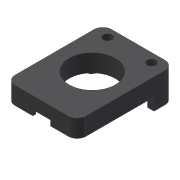
# Autodesk Inventor part: linact_palm_front
Saved by Autodesk Inventor 2014 (Build 180170000, 170)
## iProperties
Created: 2015-05-24
Part Number: linact_palm_front
Material: Generic
Document SubType Name: Modeling
Designer: Martin
Density: 1 g/cm^3
Appearance: Default
Author: Martin
Autodesk Inventor part; units mm, degrees
ref_plane "YZ Plane" through (0, 0, 0) normal (1, 0, 0) x (0, 1, 0)
ref_plane "XZ Plane" through (0, 0, 0) normal (0, 1, 0) x (-1, 0, 0)
sketch "sk_main" plane through (0, 0, 0) normal (0, 0, 1) x (1, 0, 0)
  arc A0 (-6.075, -0.5) -> (-8.075, -2.5) centre (-6.075, -2.5) ccw projected
  line L0 (-8.075, -20.5) -> (-8.075, -2.5) projected
  arc A1 (-8.075, -20.5) -> (-6.075, -22.5) centre (-6.075, -20.5) ccw projected
  line L1 (-6.075, -22.5) -> (6.075, -22.5) projected
  arc A2 (6.075, -22.5) -> (8.075, -20.5) centre (6.075, -20.5) ccw projected
  line L2 (8.075, -2.5) -> (8.075, -20.5) projected
  arc A3 (8.075, -2.5) -> (6.075, -0.5) centre (6.075, -2.5) ccw projected
  line L3 (-6.075, -0.5) -> (6.075, -0.5) projected
  circle A4 centre (-5, -2.5) radius 1 projected
  circle A5 centre (0, -20) radius 1 projected
  circle A6 centre (-5.075, -11) radius 1 projected
  circle A7 centre (5.075, -11) radius 1 projected
  circle A8 centre (5, -2.5) radius 1 projected
  circle A9 centre (0, -11) radius 3.4 projected
  circle A10 centre (0, -20) radius 2.75
  line L4 (-2, -21.8875) -> (-2, -22.5)
  line L5 (2, -21.8875) -> (2, -22.5)
  line L6 (0, 4.5828) -> (0, -27.4971) projected
  circle A11 centre (0, -11) radius 5.25
  arc A12 (-5.1545, -10.0032) -> (-5.1545, -11.9968) centre (-5.075, -11) ccw
  arc A13 (5.1545, -11.9968) -> (5.1545, -10.0032) centre (5.075, -11) ccw
  point P0 (0, 0)
  dimension "d1" = 5.5
  dimension "d2" = 4
  dimension "d3" = 10.5
  constraints: 14 point on circle, 4 centre point, 4 end point, 2 coincident, 2 concentric, 2 point on line, 1 parallel, 1 perpendicular, 1 other
  measures "d1" diameter of A10
  measures "d2" distance between parallel lines of L5 L4
  measures "d3" diameter of A11
extrude "ext_main" add sketch "sk_main" along normal blind 4 contours L3 L6 A11 A6 A10 L4 L1 A1 L0 A0 | L3 A3 L2 A2 L1 L5 A10 L6 A11 A7 | A7 A11 | A11 A6 | L4 A10 L1 | A10 L6 A5 L1 | L6 A5 A10 L1 | L1 A10 L5 picked at (5.5112, -11.1934) picked at (-5.5179, -11)
sketch "Sketch2" plane through (0, 0, 0) normal (0, 0, 1) x (1, 0, 0)
  line L0 (-6.075, -0.5) -> (6.075, -0.5) projected
  arc A0 (-6.075, -0.5) -> (-8.075, -2.5) centre (-6.075, -2.5) ccw projected
  line L1 (-8.075, -20.5) -> (-8.075, -2.5) projected
  arc A1 (8.075, -2.5) -> (6.075, -0.5) centre (6.075, -2.5) ccw projected
  line L2 (8.075, -2.5) -> (8.075, -20.5) projected
  circle A2 centre (5, -2.5) radius 1 projected
  circle A3 centre (-5, -2.5) radius 1 projected
  circle A4 centre (0, -11) radius 3.4 projected
  circle A5 centre (0, -11) radius 8.25
  line L3 (-4.0318, -2.75) -> (4.0318, -2.75)
  line L4 (-5.5309, -3.3474) -> (-8.075, -7.408)
  circle A6 centre (0, -11) radius 8.75 construction
  line L5 (5.5309, -3.3474) -> (8.075, -7.408)
  line L6 (0, 4.1) -> (0, -24.6) projected
  arc A7 (-4.0318, -2.75) -> (-5.5309, -3.3474) centre (-5, -2.5) ccw
  arc A8 (5.5309, -3.3474) -> (4.0318, -2.75) centre (5, -2.5) ccw
  line L7 (6.5663, -5) -> (8.075, -5)
  line L8 (-6.5663, -5) -> (-8.075, -5)
  point P0 (0, 0)
  dimension "d6" = 16.5
  dimension "d7" = 0.5
  dimension "d8" = 4.5
  constraints: 10 end point, 8 point on circle, 7 point on line, 4 centre point, 3 perpendicular, 2 coincident, 2 concentric, 2 symmetric about line, 2 tangent, 1 collinear
  measures "d6" diameter of A5
  measures "d7" radial gap between concentric circles of A6 A5
  measures "d8" distance between parallel lines of L0 L7
ref_plane "Work Plane1" through (-8.075, -22.5, -2.8) normal (0, 0, 1) x (1, 0, 0)
extrude "ext_base" add sketch "Sketch2" against normal up to surface (2.8 mm away) contours L0 L6 L3 A3 L4 L8 L1 A0 | L0 A1 L2 L7 L5 A2 L3 L6
sketch "Sketch4" plane through (0, 0, 0) normal (0, 0, -1) x (-1, 0, 0)
  line L0 (6.075, -22.5) -> (-6.075, -22.5) projected
  circle A0 centre (0, -20) radius 1 projected
  circle A1 centre (0, -20) radius 2.75
  line L1 (0, -27.4971) -> (0, 4.5828) projected
  line L2 (-2, -21.8875) -> (-2, -22.5)
  line L3 (2, -21.8875) -> (2, -22.5)
  point P0 (0, 0)
  dimension "d13" = 5.5
  dimension "d14" = 4
  constraints: 4 end point, 2 perpendicular, 2 point on circle, 2 point on line, 1 centre point, 1 coincident, 1 other
  measures "d13" diameter of A1
  measures "d14" distance of L3.end L2.end
extrude "ext_cut_gearhousing" cut sketch "Sketch4" against normal blind 1.2 contours L0 A1 L3 | L0 L1 A0 A1 | L0 A1 L1 A0 | L0 L2 A1
sketch "Sketch3" plane through (0, 0, 4) normal (0, 0, 1) x (1, 0, 0)
  circle A0 centre (0, -20) radius 1 projected
  point P0 (0, 0)
extrude "ext_dowelfill" add sketch "Sketch3" against normal blind 2
body "Solid1"
